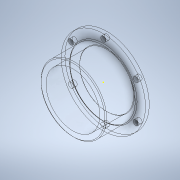
# Autodesk Inventor part: Деталь1
Saved by Autodesk Inventor 2021.2 (Build 252289000, 289)
## iProperties
Created: 2024-04-10
Part Number: Деталь1
Material: Типовые
Document SubType Name: Modeling
Designer: student
Density: 1 g/cm^3
Appearance: По умолчанию
Author: student
Autodesk Inventor part; units mm, degrees
ref_plane "YZ Plane" through (0, 0, 0) normal (1, 0, 0) x (0, 1, 0)
ref_plane "XZ Plane" through (0, 0, 0) normal (0, 1, 0) x (-1, 0, 0)
ref_plane "XY Plane" through (0, 0, 0) normal (0, 0, 1) x (1, 0, 0)
sketch "Эскиз1" plane through (0, 0, 0) normal (0, 0, 1) x (1, 0, 0)
  circle A0 centre (0, 0) radius 90
  dimension "d0" = 180
  constraints: 1 centre point, 1 coincident
  measures "d0" diameter of A0
extrude "Выдавливание1" add sketch "Эскиз1" along normal blind 8
sketch "Эскиз2" plane through (0, 0, 8) normal (0, 0, 1) x (1, 0, 0)
  point P0 (0, 0)
sketch "Эскиз3" plane through (0, 0, 0) normal (0, 0, -1) x (-1, 0, 0)
  circle A0 centre (0, 0) radius 57.5
  dimension "d3" = 115
  constraints: 1 centre point, 1 coincident
  measures "d3" diameter of A0
sketch "Эскиз4" plane through (0, 0, 8) normal (0, 0, 1) x (1, 0, 0)
  circle A0 centre (0, 0) radius 70
  dimension "d4" = 140
  constraints: 1 centre point, 1 coincident
  measures "d4" diameter of A0
extrude "Выдавливание2" add sketch "Эскиз4" along normal blind 65
hole "Отверстие1" at (0, 0, 0) direction (0, 0, 1) diameter 115 end through all
chamfer "Фаска1" distance 2 angle 45 1 edges at (-70, 0, 73)
chamfer "Фаска2" distance 1 angle 45 1 edges at (0, -57.5, 0)
fillet "Сопряжение1" radius 2 1 edges at (-70, 0, 8)
sketch "Эскиз5" plane through (0, 0, 8) normal (0, 0, 1) x (1, 0, 0)
  circle A0 centre (0, 0) radius 80
  circle A1 centre (0, 0) radius 80
  circle A2 centre (0, 0) radius 80
  circle A3 centre (0, 0) radius 80
  circle A4 centre (0, 0) radius 80
  circle A5 centre (0, 0) radius 80
  point P0 (0, 80)
  point P1 (-69.282, 40)
  point P2 (-69.282, -40)
  point P3 (0, -80)
  point P4 (69.282, -40)
  point P5 (69.282, 40)
  dimension "d21" = 160
  dimension "d24" = 360
  constraints: 2 vertical alignment, 1 coincident, 35 other
hole "Отверстие2" at (69.282, 40, 8) at (69.282, -40, 8) at (0, -80, 8) at (-69.282, -40, 8) at (-69.282, 40, 8) at (0, 80, 8) direction (0, 0, -1) diameter 11 end through all
